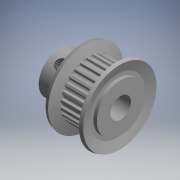
# Autodesk Inventor part: ATP26MXL025-B-P6_b
Saved by Autodesk Inventor 2017.3 (Build 213256000, 256)
## iProperties
Part Number: ATP26MXL025-B-P6_b
Material: Generic
Catalog Web Link: www.cadenas.de
Description: ATP__MXL013, ATP__MXL019, ATP__MXL025, ATP__MXL037, ATP__MXL050, BTP__MXL013, BTP__MXL019, BTP__MXL025, BTP__MXL037, BTP__MXL050, KTP__MXL013, KTP__MXL019, KTP__MXL025, KTP__MXL037, KTP__MXL050, NTP__MXL013, NTP__MXL019, NTP__MXL025, NTP__MXL037, NTP__MXL050, MTP__MXL025, MTP__MXL037, MTPB__MXL025, MTPB__MXL037, MTPP__MXL025, MTPP__MXL037, STP__MXL025, STP__MXL037_body-Timing Pulleys MXL Type
Vendor: MISUMI
Document SubType Name: Modeling
Designer: partserver
Manufacturer: MISUMI
Mass: 2.69352 g
Surface Area: 24.1533 cm^2
Volume: 2.69352 cm^3
Density: 1 g/cm^3
Appearance: PSOLRGB-192-192-192
Category: PARTsolutions
Company: MISUMI
Title: ATP26MXL025-B-P6
Author: Cadenas PARTsolutions
Comments: Timing Pulleys MXL Type
PSOL_IDENT_0: {$CADENAS_DATA\23d-libs\misumi\metric\51_timing_pulleys\mtp_mxl\atp_mxl.prj},777 {VTYP=3D},{NB=ATP26
PSOL_IDENT_1: MXL025-B-P6_b},{LINA=ATP26MXL025-B-P6},{NN=ATP__MXL013, ATP__MXL019, ATP__MXL025, ATP__MXL037, ATP__
PSOL_IDENT_2: MXL050, BTP__MXL013, BTP__MXL019, BTP__MXL025, BTP__MXL037, BTP__MXL050, KTP__MXL013, KTP__MXL019, K
PSOL_IDENT_3: TP__MXL025, KTP__MXL037, KTP__MXL050, NTP__MXL013, NTP__MXL019, NTP__MXL025, NTP__MXL037, NTP__MXL05
PSOL_IDENT_4: 0, MTP__MXL025, MTP__MXL037, MTPB__MXL025, MTPB__MXL037, MTPP__MXL025, MTPP__MXL037, STP__MXL025, ST
PSOL_IDENT_5: P__MXL037_body},{DATE=21.06.2021 00:27:39},{GEOMDATE=14.06.2021 09:50:14},{VERSION=},{LINEID=130},{W
PSOL_IDENT_6: BVAR=MATP,ST,TNW,PS,SBS,DD,Z,J,Q,R,S,T,ALT1,ALT2,M,QSC,QFC,QTC,ALT3,K,KSC,KFC,KTC,ALT4,ZM,ZSC,ZFC,ZT
PSOL_IDENT_7: C,ALT5,ALT6,ALT7,FC,ALT8,SRG,ALT9,BTC,TL,ALT10,TPC,ALT11,BC,ALT12,SLH},{WBNUMERIC=DD,Z,J,Q,R,S,T,QSC
PSOL_IDENT_8: ,QFC,QTC,K,KSC,KFC,KTC,ZSC,ZFC,ZTC,FC,SRG,BTC,TL,BC,SLH}  {NB=ATP26MXL025-B-P6_b},{LINA=ATP26MXL025-
PSOL_IDENT_9: B-P6},{KT=DUMMY},{PN=ATP26MXL025-B-P6},{TYPE=ATP},{MATP=A2017},{MATPALG= 'A2017','Aluminum Alloy 200
PSOL_IDENT_10: 0 series','S45C','1045 Carbon Steel Equivalent','SUS304','SUS304' },{ST=CA},{STALG= 'CA','Clear Anod
PSOL_IDENT_11: ize','BA','Black Anodize','HAT','Hard Clear Anodize','ENP','Electroless Nickel Plating' },{NT=26},{T
PSOL_IDENT_12: NW=MXL025},{TNWALG= 'MXL013','MXL019','MXL025','MXL037','MXL050' },{BW=6.4mm (1/4inch)},{PS=B},{PSAL
PSOL_IDENT_13: G= 'A','B' },{SBS=P},{SBSALG= 'H','Round Hole','P','Round Hole + Tap','V','Stepped Hole','F','Steppe
PSOL_IDENT_14: d Hole (Counterbore holes on the boss side)' },{DD=6.00},{DDALG=[3:4/1],4.5,[5:6/1],6.35,[7:9/1]},{D
PSOL_IDENT_15: DHA=},{DDNA=},{DDNK=[10:10/1]},{DDCA=},{DDVA=},{DDY=},{DDWB=},{DDHBK=[3:4/1],4.5,[5:6/1],6.35,[7:8/1
PSOL_IDENT_16: ]},{DDPBK=[3:4/1],4.5,[5:6/1],6.35,[7:9/1]},{DDNB=},{DDCB=},{DDVFB=[3:4/1],4.5,[5:6/1]},{Z=0},{ZALG=
PSOL_IDENT_17: [0]},{ZMIN=8.000},{ZAMAX=0.000},{ZBMAX=8.000},{DDZ=6.000},{J=0.0},{JALG=[0]},{JMIN=2.000},{JMAX=16.0
PSOL_IDENT_18: 00},{JPN=},{Q=0},{QALG=[0]},{QRMIN=8.000},{QRMAX=10},{WBQMIN=10.000},{R=0},{RALG=[0]},{WBRMAX=-2.000
PSOL_IDENT_19: },{S=0.0},{SALG=[0]},{SMAX=5.5},{T=0.0},{TALG=[0]},{TMAX=7},{SBSPN=-P6},{A=7.5},{W=11.5},{L=18.0},{P
PSOL_IDENT_20: D=16.82},{OD=16.31},{D=12},{DALG=12.000},{DE=12},{F=22},{E=14},{TT=1.0},{BBK=0.000},{TTK=0.0},{ALT1=
PSOL_IDENT_21: },{ALT1ALG= '','w/o KC90 (Set Screw Angle)','KC90','with KC90 (Set Screw Angle)' },{ANG=120.000},{AL
PSOL_IDENT_22: T1PN=},{ALT2=},{ALT2ALG= '','Not applicable' },{M=N/A},{MALG= 'N/A' },{MFTALG= 'N/A' },{MSALG= 'N/A'
PSOL_IDENT_23: },{M3D=0.000},{KDML=0.000},{ML=0.000},{MUL=0.000},{PITCH=0.000},{QSC=0.0},{QSCALG=0},{QFC=0.0},{QFC
PSOL_IDENT_24: ALG=0},{QTC=0.0},{QTCALG=0},{QPCDMIN=0.000},{QPCDMINALG=0.000},{QPCDMAX=8.000},{ALT2PN=},{TAP=0.000}
PSOL_IDENT_25: ,{ALT3=},{ALT3ALG= '','Not applicable' },{K=0.0},{KALG=0},{KMIN=4.000},{KFTMAX=0.000},{KSMAX=0.000},
PSOL_IDENT_26: {KSC=0.0},{KSCALG=0},{KFC=0.0},{KFCALG=0},{KTC=0.0},{KTCALG=0},{KSCMIN=10.000},{KPCDMIN=10.000},{KPC
PSOL_IDENT_27: DMINALG=10.000},{KPCDMAX=8.000},{ALT3PN=},{ALT4=},{ALT4ALG= '','Not applicable' },{ALT4MIN=16.500},{
PSOL_IDENT_28: ALT4MAX=3.500},{ZM=N/A},{ZMALG= 'N/A' },{ZMFTALG= 'N/A' },{ZMSALG= 'N/A' },{ZMDD1=0.0},{ZMDD2=0.0},{
PSOL_IDENT_29: ZMHH=0.0},{ZSC=0.0},{ZSCALG=[0]},{ZFC=0.0},{ZFCALG=[0]},{ZTC=0.0},{ZTCALG=[0]},{ZPCDMIN=0.000},{ZPCD
PSOL_IDENT_30: MINALG=0.000},{ZPCDMAX=8.000},{ALT4PN=},{ALT5=},{ALT5ALG= '','w/o Flange not Attached','NFC','with N
PSOL_IDENT_31: FC (Flange not Attached)' },{ALT5PN=},{ALT6=},{ALT6ALG= '','w/o Flange Attached on One Side Only','R
PSOL_IDENT_32: FC','with RFC (Flange Attached on The Boss Side Only)','LFC','with LFC (Flange Attached on The Oppos
PSOL_IDENT_33: ite Side Only)' },{ALT6PN=},{ALT7=},{ALT7ALG= '','w/o FC (Flange Cut)','FC','with FC (Flange Cut)' }
PSOL_IDENT_34: ,{FC=0.0},{FCALG=0},{FCMIN=17.5},{FCMAX=20.0},{ALT7PN=},{ALT8=},{ALT8ALG= '','Not applicable' },{ALT
PSOL_IDENT_35: 8ALGALG=8.000},{ALT8DD2=0.000},{ALT8MM=0.000},{ALT8NN=0.000},{QC=0.000},{KC=0.000},{ZC=0.000},{SRG=0
PSOL_IDENT_36: .0},{SRGALG=[0]},{SRGMAX=0.0},{SRGMAX1=0.000},{DD2=0.0},{MM=0.00},{NN=0.00},{ALT8PN=},{ALT9=},{ALT9A
PSOL_IDENT_37: LG= '','Not applicable' },{BTC9=8.000},{TL9=1.000},{BTC=0},{BTCALG=[0]},{TL=0.0},{TLALG=0},{TLMIN=1.
PSOL_IDENT_38: 000},{TLMAX=-12.000},{BTCL=0},{BTCD=0},{ALT9PN=},{WLBCTL=18.000},{ALT10=},{ALT10ALG= '','w/o TPC (Ta
PSOL_IDENT_39: pped Hole Dimension)','TPC','with TPC (Tapped Hole Dimension)' },{TPC=N/A},{TPCALG= 'N/A' },{TPCM=4.
PSOL_IDENT_40: 000},{ALT10PN=},{ALT11=},{ALT11ALG= '','Not applicable' },{BC=0.0},{BCALG=0},{BCMIN=7},{BCMAX=6},{M1
PSOL_IDENT_41: WBC=14.5},{ALT11PN=},{KTT=3},{ALT12=},{ALT12ALG= '','w/o SLH (Set Screw Length)','SLH','with SLH (Se
PSOL_IDENT_42: t Screw Length)' },{SLH=0},{SLHALG=[0]},{ALT12PN=},{AC=M4x3},{M1=4.000},{M1L=3.000},{TEDEG=20.000},{
PSOL_IDENT_43: TEB=0.670},{CD=9}
NB: ATP26MXL025-B-P6_b
NN: 0
NT: 26
NBSYN: $PN._b
LINA: ATP26MXL025-B-P6
CATALOG: Misumi
PN: ATP26MXL025-B-P6
MATP: Aluminum Alloy 2000 series
ST: Clear Anodize
TNW: MXL025
BW: 6.4mm (1/4inch)
PS: B
SBS: Round Hole + Tap
DD: 6
Z: 0
J: 0
Q: 0
R: 0
S: 0
T: 0
A: 7.5
W: 11.5
L: 18
PD: 16.82
OD: 16.31
D: 12
F: 22
E: 14
ALT1: w/o KC90 (Set Screw Angle)
ALT2: Not applicable
M: N/A
QSC: 0
QFC: 0
QTC: 0
ALT3: Not applicable
K: 0
KSC: 0
KFC: 0
KTC: 0
ALT4: Not applicable
ZM: N/A
ZMDD1: 0
ZMDD2: 0
ZMHH: 0
ZSC: 0
ZFC: 0
ZTC: 0
ALT5: w/o Flange not Attached
ALT6: w/o Flange Attached on One Side Only
ALT7: w/o FC (Flange Cut)
FC: 0
ALT8: Not applicable
SRG: 0
DD2: 0
MM: 0
ALT9: Not applicable
BTC: 0
TL: 0
BTCL: 0
BTCD: 0
ALT10: w/o TPC (Tapped Hole Dimension)
TPC: N/A
ALT11: Not applicable
BC: 0
ALT12: w/o SLH (Set Screw Length)
SLH: 0
AC: M4x3
SUPPLIER: MISUMI
ARTICLENO: ATP26MXL025-B-P6_b
BOMINFO: ATP26MXL025-B-P6
CREATOR: CADENAS GmbH
Autodesk Inventor part; units mm, degrees
note: some values were not read from the file. Chosen so that the rebuilt part matches the saved one: pattern direction of "Circular Pattern1".
sketch "_____3" plane through (0, 0, 0) normal (0, 0, 1) x (1, 0, 0)
  line L0 (18, 0) -> (0, 0)
  line L1 (0, 0) -> (0, 7)
  line L2 (0, 7) -> (1, 7)
  line L3 (1, 7) -> (1, 8.0233)
  line L4 (1, 8.0233) -> (0.2718, 10.7412)
  line L5 (0.2718, 10.7412) -> (1.2377, 11)
  line L6 (1.2377, 11) -> (2, 8.155)
  line L7 (2, 8.155) -> (9.5, 8.155)
  line L8 (9.5, 8.155) -> (10.2623, 11)
  line L9 (10.2623, 11) -> (11.2282, 10.7412)
  line L10 (11.2282, 10.7412) -> (10.5, 8.0233)
  line L11 (10.5, 8.0233) -> (10.5, 7)
  line L12 (10.5, 7) -> (11.5, 7)
  line L13 (11.5, 7) -> (11.5, 6)
  line L14 (11.5, 6) -> (18, 6)
  line L15 (18, 6) -> (18, 0)
  line L16 (18, 0) -> (0, 0)
  constraints: 34 end point
revolve "Revolution1" add sketch "_____3" angle 360 about axis through (18, 0, 0) along (1, 0, 0)
sketch "Sketch2" plane through (18, 0, 0) normal (1, 0, 0) x (0, 0, -1)
  point P0 (0, 0)
hole "Hole1" at (18, 0, 0) direction (-1, 0, 0) diameter 6 depth 18
sketch "_____6" plane through (2, 0, 0) normal (1, 0, 0) x (0, 0, -1)
  line L0 (-0.7638, 8.3752) -> (-0.7407, 8.1213)
  arc A0 (-0.5037, 7.9709) -> (-0.7407, 8.1213) centre (-0.7198, 7.8922) ccw
  line L1 (-0.5037, 7.9709) -> (-0.4092, 7.7114)
  arc A1 (-0.4092, 7.7114) -> (-0.1224, 7.514) centre (-0.1273, 7.814) ccw
  arc A2 (0.1224, 7.514) -> (-0.1224, 7.514) centre (0, 0) ccw
  arc A3 (0.1224, 7.514) -> (0.4092, 7.7114) centre (0.1273, 7.814) ccw
  line L2 (0.4092, 7.7114) -> (0.5037, 7.9709)
  arc A4 (0.7407, 8.1213) -> (0.5037, 7.9709) centre (0.7198, 7.8922) ccw
  line L3 (0.7407, 8.1213) -> (0.7638, 8.3752)
  arc A5 (0.7638, 8.3752) -> (-0.7638, 8.3752) centre (0, 0) ccw
  constraints: 12 point on circle, 8 end point, 6 centre point
extrude "Extrusion1" cut sketch "_____6" along normal blind 7.5
pattern_circular "Circular Pattern1" count 26 over 360 about axis through (2, 0, 0) along (1, 0, 0) of "Extrusion1"
sketch "_____17" plane through (14.5, 0, 0) normal (1, 0, 0) x (0, 0, -1)
  line L0 (0, 0) -> (0, 6)
  line L1 (0, 6) -> (1.621, 6)
  line L2 (1.621, 6) -> (1.621, 0)
  line L3 (1.621, 0) -> (0, 0)
  line L4 (0, 0) -> (0, 6)
  constraints: 10 end point
revolve "Revolution2" cut sketch "_____17" angle 360 about axis through (14.5, 0, 0) along (0, -1, 0)
thread "Thread1" size "M4x0.7" class "6H" standard "ISO Metric profile" length 3
sketch "_____18" plane through (14.5, 0, 0) normal (1, 0, 0) x (0, 0, -1)
  line L0 (0, 0) -> (5.1962, -3)
  line L1 (5.1962, -3) -> (4.3857, -4.4038)
  line L2 (4.3857, -4.4038) -> (-0.8105, -1.4038)
  line L3 (-0.8105, -1.4038) -> (0, 0)
  line L4 (0, 0) -> (5.1962, -3)
  constraints: 10 end point
revolve "Revolution3" cut sketch "_____18" angle 360 about axis through (14.5, 0, 0) along (0, 0.5, 0.8660254)
thread "Thread2" size "M4x0.7" class "6H" standard "ISO Metric profile" length 3
ref_plane "to_screw1_XY" through (14.5, 3, 0) normal (0, 1, 0) x (1, 0, 0)
ref_plane "to_screw1_YZ" through (14.5, 3, 0) normal (1, 0, 0) x (0, 0, -1)
ref_plane "to_screw1_ZX" through (14.5, 3, 0) normal (0, 0, -1) x (0, 1, 0)
ref_plane "to_screw2_XY" through (14.5, -1.5, -2.5981) normal (0, -0.5, -0.8660254) x (1, 0, 0)
ref_plane "to_screw2_YZ" through (14.5, -1.5, -2.5981) normal (1, 0, 0) x (0, -0.8660254, 0.5)
ref_plane "to_screw2_ZX" through (14.5, -1.5, -2.5981) normal (0, -0.8660254, 0.5) x (0, -0.5, -0.8660254)
body "Solid1"
